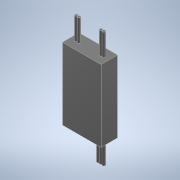
# Autodesk Inventor part: Brushed ESC
Saved by Autodesk Inventor 2022 (Build 260153000, 153)
## iProperties
Created: 2022-08-09
Part Number: Brushed ESC
Material: Generic
Document SubType Name: Modeling
Designer: Nick
Density: 1.62117 g/cm^3
Appearance: Smooth - Black
Mass: 43 g
Surface Area: 74.1149 cm^2
Volume: 26.5241 cm^3
Author: Nick
Autodesk Inventor part; units mm, degrees
ref_plane "YZ Plane" through (0, 0, 0) normal (1, 0, 0) x (0, 1, 0)
ref_plane "XZ Plane" through (0, 0, 0) normal (0, 1, 0) x (-1, 0, 0)
ref_plane "XY Plane" through (0, 0, 0) normal (0, 0, 1) x (1, 0, 0)
sketch "Sketch1" plane through (0, 0, 0) normal (0, 0, 1) x (1, 0, 0)
  line L0 (0, 0) -> (21, 0)
  line L1 (21, 0) -> (21, 39)
  line L2 (21, 39) -> (0, 39)
  line L3 (0, 39) -> (0, 0)
  dimension "d0" = 21
  dimension "d1" = 39
  constraints: 8 end point, 2 parallel, 1 horizontal, 1 perpendicular
  measures "d0" distance of L1.end L2.end
  measures "d1" distance of L0.end L1.end
extrude "Extrusion1" add sketch "Sketch1" along normal blind 9
sketch "Sketch2" plane through (21, 39, 0) normal (0, 1, 0) x (0, 0, -1)
  line L0 (0, 0) -> (-9, 0) projected
  circle A0 centre (-4.5, 3) radius 0.75
  circle A1 centre (-4.5, 4.5) radius 0.75
  circle A2 centre (-4.5, 16.5) radius 0.75
  circle A3 centre (-4.5, 18) radius 0.75
  line L1 (0, 21) -> (-9, 21) projected
  point P0 (-4.5, 0)
  point P1 (-4.5, 0)
  point P2 (-4.5, 0)
  point P3 (-4.5, 17.25)
  point P4 (-4.5, 3.75)
  dimension "d14" = 1.5
  dimension "d15" = 1.5
  dimension "d16" = 1.5
  dimension "d17" = 3
  dimension "d18" = 3
  constraints: 4 centre point, 4 vertical alignment, 3 equal radius, 2 midpoint, 1 coincident
  measures "d14" diameter of A2
  measures "d15" distance of A3.centre A2.centre
  measures "d16" distance of A1.centre A0.centre
  measures "d17" distance from line of L0 A0.centre
  measures "d18" distance from line of L1 A3.centre
extrude "Extrusion2" add sketch "Sketch2" along normal blind 12
sketch "Sketch3" plane through (0, 0, 0) normal (0, -1, 0) x (0, 0, 1)
  circle A0 centre (4.5, -18) radius 0.75
  circle A1 centre (4.5, -16.5) radius 0.75
  circle A2 centre (4.5, -15) radius 0.75
  line L0 (0, -21) -> (9, -21) projected
  point P0 (4.5, -21)
  point P1 (4.5, -15.75)
  point P2 (4.5, -17.25)
  dimension "d19" = 1.5
  dimension "d20" = 1.5
  dimension "d21" = 1.5
  dimension "d22" = 3
  constraints: 3 centre point, 3 vertical alignment, 2 equal radius, 1 midpoint
  measures "d19" diameter of A1
  measures "d20" distance of A2.centre A1.centre
  measures "d21" distance of A0.centre A1.centre
  measures "d22" distance from line of L0 A0.centre
extrude "Extrusion3" add sketch "Sketch3" along normal blind 12
equation "\"d21\" = d20"
body "Solid1"
